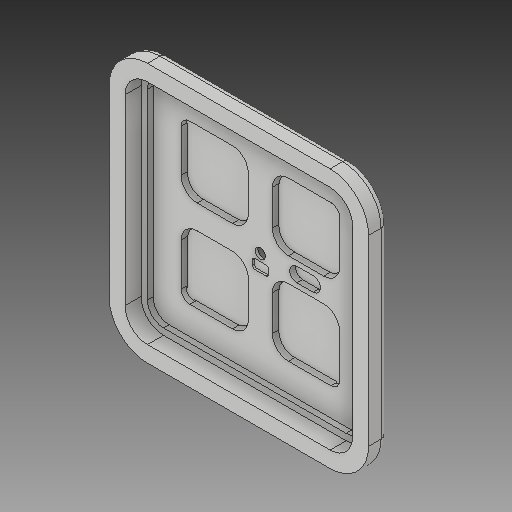
# Autodesk Inventor part: V4
Saved by Autodesk Inventor 2020 (Build 240168000, 168)
## iProperties
Created: 2020-01-08
Part Number: V4
Material: Generic
Document SubType Name: Modeling
Designer: user
Density: 1 g/cm^3
Appearance: Default
Author: user
Autodesk Inventor part; units mm, degrees
ref_plane "YZ Plane" through (0, 0, 0) normal (1, 0, 0) x (0, 1, 0)
ref_plane "XZ Plane" through (0, 0, 0) normal (0, 1, 0) x (-1, 0, 0)
ref_plane "XY Plane" through (0, 0, 0) normal (0, 0, 1) x (1, 0, 0)
sketch "Sketch1" plane through (0, 0, 0) normal (0, 0, 1) x (1, 0, 0)
  line L0 (-28.5, 40.5) -> (28.5, 40.5)
  line L1 (40.5, 28.5) -> (40.5, -28.5)
  line L2 (28.5, -40.5) -> (-28.5, -40.5)
  line L3 (-40.5, -28.5) -> (-40.5, 28.5)
  arc A0 (-28.5, 40.5) -> (-40.5, 28.5) centre (-28.5, 28.5) ccw
  arc A1 (40.5, 28.5) -> (28.5, 40.5) centre (28.5, 28.5) ccw
  arc A2 (28.5, -40.5) -> (40.5, -28.5) centre (28.5, -28.5) ccw
  arc A3 (-40.5, -28.5) -> (-28.5, -40.5) centre (-28.5, -28.5) ccw
  line L4 (-28.5, 28.5) -> (28.5, -28.5) construction
  point P0 (0, 0)
  point P1 (0, 0)
  dimension "d0" = 12
  dimension "d1" = 81
  dimension "d40" = 81
  constraints: 10 end point, 8 point on circle, 8 tangent, 4 centre point, 3 equal radius, 2 parallel, 1 coincident, 1 horizontal, 1 midpoint, 1 perpendicular
  measures "d0" radius of A0
  measures "d1" distance between parallel lines of L2 L0
  measures "d40" distance between parallel lines of L1 L3
extrude "Extrusion1" add sketch "Sketch1" along normal blind 10.25
sketch "Sketch2" plane through (0, 0, 10.25) normal (0, 0, 1) x (1, 0, 0)
  line L0 (28.5, 40.5) -> (-28.5, 40.5) construction
  arc A0 (-28.5, 40.5) -> (-40.5, 28.5) centre (-28.5, 28.5) ccw construction
  line L1 (-40.5, 28.5) -> (-40.5, -28.5) construction
  arc A1 (-40.5, -28.5) -> (-28.5, -40.5) centre (-28.5, -28.5) ccw construction
  line L2 (-28.5, -40.5) -> (28.5, -40.5) construction
  arc A2 (28.5, -40.5) -> (40.5, -28.5) centre (28.5, -28.5) ccw construction
  line L3 (40.5, -28.5) -> (40.5, 28.5) construction
  arc A3 (40.5, 28.5) -> (28.5, 40.5) centre (28.5, 28.5) ccw construction
  line L4 (-28.5, 35.5) -> (28.5, 35.5)
  arc A4 (35.5, 28.5) -> (28.5, 35.5) centre (28.5, 28.5) ccw
  line L5 (35.5, 28.5) -> (35.5, -28.5)
  arc A5 (28.5, -35.5) -> (35.5, -28.5) centre (28.5, -28.5) ccw
  line L6 (28.5, -35.5) -> (-28.5, -35.5)
  arc A6 (-35.5, -28.5) -> (-28.5, -35.5) centre (-28.5, -28.5) ccw
  line L7 (-35.5, -28.5) -> (-35.5, 28.5)
  arc A7 (-28.5, 35.5) -> (-35.5, 28.5) centre (-28.5, 28.5) ccw
  point P0 (0, 0)
  dimension "d4" = 5
  constraints: 8 end point, 8 point on circle, 4 centre point, 7 other
  measures "d4" distance between parallel lines of L1 L7
extrude "Extrusion2" cut sketch "Sketch2" against normal blind 5
sketch "Sketch3" plane through (0, 0, 5.25) normal (0, 0, 1) x (1, 0, 0)
  line L0 (-28.5, 35.5) -> (28.5, 35.5) construction
  arc A0 (-28.5, 35.5) -> (-35.5, 28.5) centre (-28.5, 28.5) ccw construction
  line L1 (-35.5, -28.5) -> (-35.5, 28.5) construction
  arc A1 (-35.5, -28.5) -> (-28.5, -35.5) centre (-28.5, -28.5) ccw construction
  line L2 (28.5, -35.5) -> (-28.5, -35.5) construction
  arc A2 (28.5, -35.5) -> (35.5, -28.5) centre (28.5, -28.5) ccw construction
  line L3 (35.5, 28.5) -> (35.5, -28.5) construction
  arc A3 (35.5, 28.5) -> (28.5, 35.5) centre (28.5, 28.5) ccw construction
  line L4 (28.5, 33.5) -> (-28.5, 33.5)
  arc A4 (-28.5, 33.5) -> (-33.5, 28.5) centre (-28.5, 28.5) ccw
  line L5 (-33.5, 28.5) -> (-33.5, -28.5)
  arc A5 (-33.5, -28.5) -> (-28.5, -33.5) centre (-28.5, -28.5) ccw
  line L6 (-28.5, -33.5) -> (28.5, -33.5)
  arc A6 (28.5, -33.5) -> (33.5, -28.5) centre (28.5, -28.5) ccw
  line L7 (33.5, -28.5) -> (33.5, 28.5)
  arc A7 (33.5, 28.5) -> (28.5, 33.5) centre (28.5, 28.5) ccw
  point P0 (0, 0)
  dimension "d7" = 2
  constraints: 8 end point, 8 point on circle, 4 centre point, 7 other
  measures "d7" distance between parallel lines of L0 L4
extrude "Extrusion3" cut sketch "Sketch3" against normal blind 1.75
chamfer "Chamfer1" distance 9 angle 30 8 edges at (0, 40.5, 0) (36.9853, 36.9853, 0) (40.5, 0, 0) (36.9853, -36.9853, 0) (0, -40.5, 0) (-36.9853, -36.9853, 0) (-40.5, 0, 0) (-36.9853, 36.9853, 0) measured on face at (40, 0, 0) measured on face at (-36.6317, -36.6317, 0) measured on face at (0, 40, 0) measured on face at (0, -40, 0) measured on face at (-36.6317, 36.6317, 0) measured on face at (36.6317, 36.6317, 0) measured on face at (-40, 0, 0) measured on face at (36.6317, -36.6317, 0)
sketch "Sketch5" plane through (0, 0, 0) normal (0, 0, -1) x (-1, 0, 0)
  line L0 (-8.75, 3.75) -> (-19.75, 3.75)
  line L1 (-24.75, 8.75) -> (-24.75, 22.0251)
  line L2 (-22.0251, 24.75) -> (-8.75, 24.75)
  line L3 (-3.75, 19.75) -> (-3.75, 8.75)
  arc A0 (-24.75, 8.75) -> (-19.75, 3.75) centre (-19.75, 8.75) ccw
  arc A1 (-3.75, 19.75) -> (-8.75, 24.75) centre (-8.75, 19.75) ccw
  arc A2 (-8.75, 3.75) -> (-3.75, 8.75) centre (-8.75, 8.75) ccw
  line L4 (17.252, -17.252) -> (-8.75, 8.75) construction
  line L5 (-8.75, 24.25) -> (-22.0251, 24.25)
  line L6 (-24.25, 22.0251) -> (-24.25, 8.75)
  arc A3 (-24.25, 8.75) -> (-19.75, 4.25) centre (-19.75, 8.75) ccw
  line L7 (-19.75, 4.25) -> (-8.75, 4.25)
  arc A4 (-8.75, 4.25) -> (-4.25, 8.75) centre (-8.75, 8.75) ccw
  line L8 (-4.25, 8.75) -> (-4.25, 19.75)
  arc A5 (-4.25, 19.75) -> (-8.75, 24.25) centre (-8.75, 19.75) ccw
  line L9 (-45.752, 45.752) -> (-19.75, 19.75) construction
  line L10 (-8.75, 24.25) -> (-8.75, 4.25) construction
  line L11 (-24.25, 8.75) -> (-4.25, 8.75) construction
  line L12 (-8.75, 24.25) -> (-8.75, 24.75) construction
  line L13 (-24.25, 8.75) -> (-24.75, 8.75) construction
  line L14 (-8.75, 19.75) -> (-19.75, 19.75) construction
  line L15 (-19.75, 8.75) -> (-19.75, 19.75) construction
  arc A6 (-22.2751, 24.5) -> (-22.0251, 24.25) centre (-22.0251, 24.5) ccw
  arc A7 (-22.0251, 24.75) -> (-22.2751, 24.5) centre (-22.0251, 24.5) ccw
  arc A8 (-24.25, 22.0251) -> (-24.5, 21.7751) centre (-24.5, 22.0251) ccw construction
  arc A9 (-24.5, 21.7751) -> (-24.75, 22.0251) centre (-24.5, 22.0251) ccw construction
  line L16 (-23.2626, 23.2626) -> (-22.2019, 24.3232) construction
  line L17 (-23.2626, 23.2626) -> (-24.3232, 22.2019) construction
  arc A10 (-28.5, 31.5) -> (-31.5, 28.5) centre (-28.5, 28.5) ccw construction
  arc A11 (-24.25, 22.0251) -> (-24.75, 22.0251) centre (-24.5, 22.0251) ccw
  line L18 (-3.75, -8.75) -> (-3.75, -19.75)
  line L19 (-8.75, -4.25) -> (-19.75, -4.25)
  line L20 (-4.25, -19.75) -> (-4.25, -8.75)
  line L21 (-24.25, -8.75) -> (-4.25, -8.75) construction
  line L22 (-8.75, -24.25) -> (-8.75, -4.25) construction
  arc A12 (-19.75, -4.25) -> (-24.25, -8.75) centre (-19.75, -8.75) ccw
  line L23 (-8.75, -19.75) -> (-19.75, -19.75) construction
  line L24 (-19.75, -8.75) -> (-19.75, -19.75) construction
  line L25 (-23.2626, -23.2626) -> (-22.2019, -24.3232) construction
  line L26 (-24.25, -8.75) -> (-24.25, -22.0251)
  line L27 (-24.75, -22.0251) -> (-24.75, -8.75)
  line L28 (-24.25, -8.75) -> (-24.75, -8.75) construction
  arc A13 (-19.75, -3.75) -> (-24.75, -8.75) centre (-19.75, -8.75) ccw
  line L29 (-19.75, -3.75) -> (-8.75, -3.75)
  arc A14 (-3.75, -8.75) -> (-8.75, -3.75) centre (-8.75, -8.75) ccw
  arc A15 (-4.25, -8.75) -> (-8.75, -4.25) centre (-8.75, -8.75) ccw
  line L30 (-8.75, -24.75) -> (-22.0251, -24.75)
  line L31 (-22.0251, -24.25) -> (-8.75, -24.25)
  line L32 (-8.75, -24.25) -> (-8.75, -24.75) construction
  arc A16 (-8.75, -24.25) -> (-4.25, -19.75) centre (-8.75, -19.75) ccw
  arc A17 (-8.75, -24.75) -> (-3.75, -19.75) centre (-8.75, -19.75) ccw
  arc A18 (-24.75, -22.0251) -> (-24.5, -22.2751) centre (-24.5, -22.0251) ccw
  arc A19 (-24.5, -22.2751) -> (-24.25, -22.0251) centre (-24.5, -22.0251) ccw
  line L33 (-23.2626, -23.2626) -> (-24.3232, -22.2019) construction
  arc A20 (-21.7751, -24.5) -> (-22.0251, -24.75) centre (-22.0251, -24.5) ccw construction
  arc A21 (-22.0251, -24.25) -> (-21.7751, -24.5) centre (-22.0251, -24.5) ccw construction
  arc A22 (-22.0251, -24.25) -> (-22.0251, -24.75) centre (-22.0251, -24.5) ccw
  line L34 (8.75, -3.75) -> (19.75, -3.75)
  line L35 (4.25, -8.75) -> (4.25, -19.75)
  line L36 (19.75, -4.25) -> (8.75, -4.25)
  line L37 (8.75, -24.25) -> (8.75, -4.25) construction
  line L38 (24.25, -8.75) -> (4.25, -8.75) construction
  arc A23 (4.25, -19.75) -> (8.75, -24.25) centre (8.75, -19.75) ccw
  line L39 (19.75, -8.75) -> (19.75, -19.75) construction
  line L40 (8.75, -19.75) -> (19.75, -19.75) construction
  line L41 (23.2626, -23.2626) -> (24.3232, -22.2019) construction
  line L42 (8.75, -24.25) -> (22.0251, -24.25)
  line L43 (22.0251, -24.75) -> (8.75, -24.75)
  line L44 (8.75, -24.25) -> (8.75, -24.75) construction
  arc A24 (3.75, -19.75) -> (8.75, -24.75) centre (8.75, -19.75) ccw
  line L45 (3.75, -19.75) -> (3.75, -8.75)
  arc A25 (8.75, -3.75) -> (3.75, -8.75) centre (8.75, -8.75) ccw
  arc A26 (8.75, -4.25) -> (4.25, -8.75) centre (8.75, -8.75) ccw
  line L46 (24.75, -8.75) -> (24.75, -22.0251)
  line L47 (24.25, -22.0251) -> (24.25, -8.75)
  line L48 (24.25, -8.75) -> (24.75, -8.75) construction
  arc A27 (24.25, -8.75) -> (19.75, -4.25) centre (19.75, -8.75) ccw
  arc A28 (24.75, -8.75) -> (19.75, -3.75) centre (19.75, -8.75) ccw
  arc A29 (22.0251, -24.75) -> (22.2751, -24.5) centre (22.0251, -24.5) ccw
  arc A30 (22.2751, -24.5) -> (22.0251, -24.25) centre (22.0251, -24.5) ccw
  line L49 (23.2626, -23.2626) -> (22.2019, -24.3232) construction
  arc A31 (24.5, -21.7751) -> (24.75, -22.0251) centre (24.5, -22.0251) ccw construction
  arc A32 (24.25, -22.0251) -> (24.5, -21.7751) centre (24.5, -22.0251) ccw construction
  arc A33 (24.25, -22.0251) -> (24.75, -22.0251) centre (24.5, -22.0251) ccw
  line L50 (3.75, 8.75) -> (3.75, 19.75)
  line L51 (8.75, 4.25) -> (19.75, 4.25)
  line L52 (4.25, 19.75) -> (4.25, 8.75)
  line L53 (24.25, 8.75) -> (4.25, 8.75) construction
  line L54 (8.75, 24.25) -> (8.75, 4.25) construction
  arc A34 (19.75, 4.25) -> (24.25, 8.75) centre (19.75, 8.75) ccw
  line L55 (8.75, 19.75) -> (19.75, 19.75) construction
  line L56 (19.75, 8.75) -> (19.75, 19.75) construction
  line L57 (23.2626, 23.2626) -> (22.2019, 24.3232) construction
  line L58 (24.25, 8.75) -> (24.25, 22.0251)
  line L59 (24.75, 22.0251) -> (24.75, 8.75)
  line L60 (24.25, 8.75) -> (24.75, 8.75) construction
  arc A35 (19.75, 3.75) -> (24.75, 8.75) centre (19.75, 8.75) ccw
  line L61 (19.75, 3.75) -> (8.75, 3.75)
  arc A36 (3.75, 8.75) -> (8.75, 3.75) centre (8.75, 8.75) ccw
  arc A37 (4.25, 8.75) -> (8.75, 4.25) centre (8.75, 8.75) ccw
  line L62 (8.75, 24.75) -> (22.0251, 24.75)
  line L63 (22.0251, 24.25) -> (8.75, 24.25)
  line L64 (8.75, 24.25) -> (8.75, 24.75) construction
  arc A38 (8.75, 24.25) -> (4.25, 19.75) centre (8.75, 19.75) ccw
  arc A39 (8.75, 24.75) -> (3.75, 19.75) centre (8.75, 19.75) ccw
  arc A40 (24.75, 22.0251) -> (24.5, 22.2751) centre (24.5, 22.0251) ccw
  arc A41 (24.5, 22.2751) -> (24.25, 22.0251) centre (24.5, 22.0251) ccw
  line L65 (23.2626, 23.2626) -> (24.3232, 22.2019) construction
  arc A42 (21.7751, 24.5) -> (22.0251, 24.75) centre (22.0251, 24.5) ccw construction
  arc A43 (22.0251, 24.25) -> (21.7751, 24.5) centre (22.0251, 24.5) ccw construction
  arc A44 (22.0251, 24.25) -> (22.0251, 24.75) centre (22.0251, 24.5) ccw
  line L66 (0, 0) -> (0, 0)
  line L67 (24.75, -15.3876) -> (31.5, -15.3876) construction
  line L68 (31.5, 28.5) -> (31.5, -28.5) construction
  line L69 (15.3876, -24.75) -> (15.3876, -31.5) construction
  line L70 (28.5, -31.5) -> (-28.5, -31.5) construction
  point P0 (-22.2751, 24.75)
  point P1 (-24.75, 21.7751)
  point P2 (-24.25, 21.7751)
  point P3 (-22.2751, 24.25)
  point P4 (-24.25, -22.2751)
  point P5 (-24.75, -22.2751)
  point P6 (-21.7751, -24.75)
  point P7 (-21.7751, -24.25)
  point P8 (22.2751, -24.25)
  point P9 (22.2751, -24.75)
  point P10 (24.75, -21.7751)
  point P11 (24.25, -21.7751)
  point P12 (24.25, 22.2751)
  point P13 (24.75, 22.2751)
  point P14 (21.7751, 24.75)
  point P15 (21.7751, 24.25)
  dimension "d23" = 0.5
  dimension "d24" = 5
  dimension "d25" = 20
  dimension "d26" = 0.25
  dimension "d27" = 3
  dimension "d32" = 360
  dimension "d41" = 7.5
  constraints: 138 end point, 96 point on circle, 44 centre point, 27 point on line, 11 tangent, 7 perpendicular, 6 equal length, 4 horizontal, 4 parallel, 3 collinear, 3 equal radius, 2 midpoint, 2 vertical, 1 coincident, 315 other
  measures "d23" distance between parallel lines of L0 L7
  measures "d24" radius of A0
  measures "d25" distance between parallel lines of L8 L6
  measures "d26" radius of A6
  measures "d27" distance of L17.end L16.end
  measures "d41" distance between parallel lines of L50 L3
extrude "Extrusion4" cut sketch "Sketch5" against normal through all
fillet "Fillet2" radius 2 16 edges at (36.9853, 36.9853, 5.1962) (40.5, 0, 5.1962) (36.9853, -36.9853, 5.1962) (0, -40.5, 5.1962) (-36.9853, -36.9853, 5.1962) (-40.5, 0, 5.1962) (-36.9853, 36.9853, 5.1962) (0, 40.5, 5.1962) (-30.6213, 30.6213, 0) (-31.5, 0, 0) (-30.6213, -30.6213, 0) (0, -31.5, 0) (30.6213, -30.6213, 0) (31.5, 0, 0) (30.6213, 30.6213, 0) (0, 31.5, 0)
sketch "Sketch7" plane through (0, 0, 3.5) normal (0, 0, 1) x (1, 0, 0)
  line L0 (-3.75, -8.75) -> (-3.75, -19.75) projected
  arc A0 (-8.75, -24.75) -> (-3.75, -19.75) centre (-8.75, -19.75) ccw projected
  line L1 (-8.75, -24.75) -> (-22.0251, -24.75) projected
  arc A1 (-22.0251, -24.25) -> (-22.0251, -24.75) centre (-22.0251, -24.5) ccw projected
  line L2 (-22.0251, -24.25) -> (-8.75, -24.25) projected
  arc A2 (-8.75, -24.25) -> (-4.25, -19.75) centre (-8.75, -19.75) ccw projected
  line L3 (-4.25, -19.75) -> (-4.25, -8.75) projected
  arc A3 (-4.25, -8.75) -> (-8.75, -4.25) centre (-8.75, -8.75) ccw projected
  line L4 (-8.75, -4.25) -> (-19.75, -4.25) projected
  arc A4 (-19.75, -4.25) -> (-24.25, -8.75) centre (-19.75, -8.75) ccw projected
  line L5 (-24.25, -8.75) -> (-24.25, -22.0251) projected
  arc A5 (-24.75, -22.0251) -> (-24.25, -22.0251) centre (-24.5, -22.0251) ccw projected
  line L6 (-24.75, -22.0251) -> (-24.75, -8.75) projected
  arc A6 (-19.75, -3.75) -> (-24.75, -8.75) centre (-19.75, -8.75) ccw projected
  line L7 (-19.75, -3.75) -> (-8.75, -3.75) projected
  arc A7 (-3.75, -8.75) -> (-8.75, -3.75) centre (-8.75, -8.75) ccw projected
  line L8 (22.0251, 24.25) -> (8.75, 24.25) projected
  arc A8 (8.75, 24.25) -> (4.25, 19.75) centre (8.75, 19.75) ccw projected
  line L9 (4.25, 19.75) -> (4.25, 8.75) projected
  arc A9 (4.25, 8.75) -> (8.75, 4.25) centre (8.75, 8.75) ccw projected
  line L10 (8.75, 4.25) -> (19.75, 4.25) projected
  arc A10 (19.75, 4.25) -> (24.25, 8.75) centre (19.75, 8.75) ccw projected
  line L11 (24.25, 8.75) -> (24.25, 22.0251) projected
  arc A11 (24.75, 22.0251) -> (24.25, 22.0251) centre (24.5, 22.0251) ccw projected
  line L12 (24.75, 22.0251) -> (24.75, 8.75) projected
  arc A12 (19.75, 3.75) -> (24.75, 8.75) centre (19.75, 8.75) ccw projected
  line L13 (19.75, 3.75) -> (8.75, 3.75) projected
  arc A13 (3.75, 8.75) -> (8.75, 3.75) centre (8.75, 8.75) ccw projected
  line L14 (3.75, 8.75) -> (3.75, 19.75) projected
  arc A14 (8.75, 24.75) -> (3.75, 19.75) centre (8.75, 19.75) ccw projected
  line L15 (8.75, 24.75) -> (22.0251, 24.75) projected
  arc A15 (22.0251, 24.25) -> (22.0251, 24.75) centre (22.0251, 24.5) ccw projected
  line L16 (8.75, -3.75) -> (19.75, -3.75) projected
  arc A16 (24.75, -8.75) -> (19.75, -3.75) centre (19.75, -8.75) ccw projected
  line L17 (24.75, -8.75) -> (24.75, -22.0251) projected
  arc A17 (24.25, -22.0251) -> (24.75, -22.0251) centre (24.5, -22.0251) ccw projected
  line L18 (24.25, -22.0251) -> (24.25, -8.75) projected
  arc A18 (24.25, -8.75) -> (19.75, -4.25) centre (19.75, -8.75) ccw projected
  line L19 (19.75, -4.25) -> (8.75, -4.25) projected
  arc A19 (8.75, -4.25) -> (4.25, -8.75) centre (8.75, -8.75) ccw projected
  line L20 (4.25, -8.75) -> (4.25, -19.75) projected
  arc A20 (4.25, -19.75) -> (8.75, -24.25) centre (8.75, -19.75) ccw projected
  line L21 (8.75, -24.25) -> (22.0251, -24.25) projected
  arc A21 (22.0251, -24.75) -> (22.0251, -24.25) centre (22.0251, -24.5) ccw projected
  line L22 (22.0251, -24.75) -> (8.75, -24.75) projected
  arc A22 (3.75, -19.75) -> (8.75, -24.75) centre (8.75, -19.75) ccw projected
  line L23 (3.75, -19.75) -> (3.75, -8.75) projected
  arc A23 (8.75, -3.75) -> (3.75, -8.75) centre (8.75, -8.75) ccw projected
  line L24 (-8.75, 3.75) -> (-19.75, 3.75) projected
  arc A24 (-24.75, 8.75) -> (-19.75, 3.75) centre (-19.75, 8.75) ccw projected
  line L25 (-24.75, 8.75) -> (-24.75, 22.0251) projected
  arc A25 (-24.25, 22.0251) -> (-24.75, 22.0251) centre (-24.5, 22.0251) ccw projected
  line L26 (-24.25, 22.0251) -> (-24.25, 8.75) projected
  arc A26 (-24.25, 8.75) -> (-19.75, 4.25) centre (-19.75, 8.75) ccw projected
  line L27 (-19.75, 4.25) -> (-8.75, 4.25) projected
  arc A27 (-8.75, 4.25) -> (-4.25, 8.75) centre (-8.75, 8.75) ccw projected
  line L28 (-4.25, 8.75) -> (-4.25, 19.75) projected
  arc A28 (-4.25, 19.75) -> (-8.75, 24.25) centre (-8.75, 19.75) ccw projected
  line L29 (-8.75, 24.25) -> (-22.0251, 24.25) projected
  arc A29 (-22.0251, 24.75) -> (-22.0251, 24.25) centre (-22.0251, 24.5) ccw projected
  line L30 (-22.0251, 24.75) -> (-8.75, 24.75) projected
  arc A30 (-3.75, 19.75) -> (-8.75, 24.75) centre (-8.75, 19.75) ccw projected
  line L31 (-3.75, 19.75) -> (-3.75, 8.75) projected
  arc A31 (-8.75, 3.75) -> (-3.75, 8.75) centre (-8.75, 8.75) ccw projected
  line L32 (-28.5, 33.5) -> (28.5, 33.5) projected
  arc A32 (-28.5, 33.5) -> (-33.5, 28.5) centre (-28.5, 28.5) ccw projected
  line L33 (-33.5, -28.5) -> (-33.5, 28.5) projected
  arc A33 (-33.5, -28.5) -> (-28.5, -33.5) centre (-28.5, -28.5) ccw projected
  line L34 (28.5, -33.5) -> (-28.5, -33.5) projected
  arc A34 (28.5, -33.5) -> (33.5, -28.5) centre (28.5, -28.5) ccw projected
  line L35 (33.5, 28.5) -> (33.5, -28.5) projected
  arc A35 (33.5, 28.5) -> (28.5, 33.5) centre (28.5, 28.5) ccw projected
  arc A36 (-24.75, -22.0251) -> (-22.0251, -24.75) centre (-22.0251, -22.0251) ccw
  arc A37 (-22.0251, 24.75) -> (-24.75, 22.0251) centre (-22.0251, 22.0251) ccw
  arc A38 (22.0251, 24.25) -> (22.0251, 24.75) centre (22.0251, 24.5) ccw projected
  arc A39 (24.75, 22.0251) -> (22.0251, 24.75) centre (22.0251, 22.0251) ccw
  line L36 (22.0251, -24.75) -> (8.75, -24.75) projected
  arc A40 (22.0251, -24.75) -> (24.75, -22.0251) centre (22.0251, -22.0251) ccw
  point P0 (0, 0)
  constraints: 8 point on circle, 4 centre point, 4 tangent
extrude "Extrusion6" cut sketch "Sketch7" against normal blind 1.5 contours L0 A0 L1 A1 L2 A2 L3 A3 L4 A4 L5 A5 L6 A6 L7 A7 | A36 A5 L5 A4 L4 A3 L3 A2 L2 A1 | A15 A39 A11 L11 A10 L10 A9 L9 A8 L8 | L8 A8 L9 A9 L10 A10 L11 A11 L12 A12 L13 A13 L14 A14 L15 A15 | L16 A16 L17 A17 L18 A18 L19 A19 L20 A20 L21 A21 L22 A22 L23 A23 | A40 A21 L21 A20 L20 A19 L19 A18 L18 A17 | L24 A24 L25 A25 L26 A26 L27 A27 L28 A28 L29 A29 L30 A30 L31 A31 | A37 A29 L29 A28 L28 A27 L27 A26 L26 A25
sketch "Sketch8" plane through (0, 0, 0) normal (0, 0, -1) x (-1, 0, 0)
  arc A0 (8.75, -4.25) -> (4.25, -8.75) centre (8.75, -8.75) ccw construction
  arc A1 (-8.75, 4.25) -> (-4.25, 8.75) centre (-8.75, 8.75) ccw construction
  line L0 (8.75, -8.75) -> (-8.75, 8.75) construction
  point P0 (0, 0)
  point P1 (0, 0)
  constraints: 2 end point, 1 midpoint
hole "Hole1" at (0, 0, 0) direction (0, 0, 1) diameter 3.2 end through all counterbore diameter 5.7 counterbore depth 2.7
sketch "Sketch10" plane through (0, 0, 3.5) normal (0, 0, 1) x (1, 0, 0)
  line L0 (2.5, -4.461) -> (2.5, -2.961)
  line L1 (1.75, -2.211) -> (-1.75, -2.211)
  line L2 (-2.5, -2.961) -> (-2.5, -4.461)
  line L3 (-1.75, -5.211) -> (1.75, -5.211)
  line L4 (16.4884, 0) -> (11.4084, 0) construction
  line L5 (16.4884, 2.25) -> (11.4084, 2.25)
  line L6 (11.4084, -2.25) -> (16.4884, -2.25)
  arc A0 (16.4884, -2.25) -> (16.4884, 2.25) centre (16.4884, 0) ccw
  arc A1 (11.4084, 2.25) -> (11.4084, -2.25) centre (11.4084, 0) ccw
  circle A2 centre (0, 0) radius 1.6 construction
  line L7 (13.9484, -2.25) -> (13.9484, -3.75) construction
  line L8 (8.75, -3.75) -> (19.75, -3.75) construction
  line L9 (13.9484, 2.25) -> (13.9484, 3.75) construction
  line L10 (8.75, 3.75) -> (19.75, 3.75) construction
  arc A3 (-2.5, -4.461) -> (-1.75, -5.211) centre (-1.75, -4.461) ccw
  arc A4 (1.75, -5.211) -> (2.5, -4.461) centre (1.75, -4.461) ccw
  arc A5 (2.5, -2.961) -> (1.75, -2.211) centre (1.75, -2.961) ccw
  arc A6 (-1.75, -2.211) -> (-2.5, -2.961) centre (-1.75, -2.961) ccw
  line L11 (1.75, -4.461) -> (0, 0) construction
  line L12 (0, 0) -> (-1.75, -4.461) construction
  point P0 (2.5, -5.211)
  point P1 (-2.5, -2.211)
  point P2 (-2.5, -5.211)
  point P3 (13.9484, 0)
  dimension "d70" = 5
  dimension "d71" = 3
  dimension "d73" = 5.08
  dimension "d76" = 0.75
  dimension "d84" = 13.9484
  dimension "d85" = 2.211
  dimension "d86" = 4.5
  constraints: 24 end point, 12 point on circle, 12 tangent, 9 point on line, 6 centre point, 3 equal radius, 3 midpoint, 3 parallel, 2 equal length, 2 horizontal, 2 vertical, 1 coincident, 1 perpendicular
  measures "d70" distance of point (-2.5, -5.211) point (2.5, -5.211)
  measures "d71" distance of point (-2.5, -2.211) point (-2.5, -5.211)
  measures "d73" distance of L5.start L5.end
  measures "d76" radius of A3
  measures "d84" distance of L11.end point (13.948, 0)
  measures "d85" distance from line of L11.end L1
  measures "d86" distance between parallel lines of L5 L6
extrude "Extrusion7" cut sketch "Sketch10" against normal blind 0.64 contours A4 L3 A3 L2 A6 L1 A5 L0
extrude "Extrusion8" cut sketch "Sketch10" against normal blind 1.75 contours A0 L6 A1 L5
sketch "Sketch9" plane through (0, 0, 0) normal (0, 0, -1) x (-1, 0, 0)
  arc A0 (-4.25, 19.75) -> (-8.75, 24.25) centre (-8.75, 19.75) ccw construction
  circle A1 centre (0, 0) radius 1.6 construction
  arc A2 (-24.25, 8.75) -> (-19.75, 4.25) centre (-19.75, 8.75) ccw construction
  line L0 (-8.75, 19.75) -> (-19.75, 8.75) construction
  circle A3 centre (-14.25, 14.25) radius 2
  circle A4 centre (-17.0784, 11.4216) radius 2
  circle A5 centre (-16.25, 10.7859) radius 2
  circle A6 centre (-15.2853, 10.3863) radius 2
  circle A7 centre (-14.25, 10.25) radius 2
  circle A8 centre (-13.2147, 10.3863) radius 2
  circle A9 centre (-12.25, 10.7859) radius 2
  circle A10 centre (-11.4216, 11.4216) radius 2
  circle A11 centre (-10.7859, 12.25) radius 2
  circle A12 centre (-10.3863, 13.2147) radius 2
  circle A13 centre (-10.25, 14.25) radius 2
  circle A14 centre (-10.3863, 15.2853) radius 2
  circle A15 centre (-10.7859, 16.25) radius 2
  circle A16 centre (-11.4216, 17.0784) radius 2
  circle A17 centre (-12.25, 17.7141) radius 2
  circle A18 centre (-13.2147, 18.1137) radius 2
  circle A19 centre (-14.25, 18.25) radius 2
  circle A20 centre (-15.2853, 18.1137) radius 2
  circle A21 centre (-16.25, 17.7141) radius 2
  circle A22 centre (-17.0784, 17.0784) radius 2
  circle A23 centre (-17.7141, 16.25) radius 2
  circle A24 centre (-18.1137, 15.2853) radius 2
  circle A25 centre (-18.25, 14.25) radius 2
  circle A26 centre (-18.1137, 13.2147) radius 2
  circle A27 centre (-17.7141, 12.25) radius 2
  circle A28 centre (-10.7859, -12.25) radius 2
  circle A29 centre (-10.3863, -13.2147) radius 2
  circle A30 centre (-10.3863, -15.2853) radius 2
  circle A31 centre (-10.7859, -16.25) radius 2
  circle A32 centre (-10.25, -14.25) radius 2
  circle A33 centre (-18.1137, -13.2147) radius 2
  circle A34 centre (-18.25, -14.25) radius 2
  circle A35 centre (-18.1137, -15.2853) radius 2
  circle A36 centre (-14.25, -18.25) radius 2
  circle A37 centre (-15.2853, -18.1137) radius 2
  circle A38 centre (-17.7141, -16.25) radius 2
  circle A39 centre (-17.0784, -17.0784) radius 2
  circle A40 centre (-16.25, -17.7141) radius 2
  circle A41 centre (-11.4216, -11.4216) radius 2
  circle A42 centre (-12.25, -10.7859) radius 2
  line L1 (-19.75, -8.75) -> (-8.75, -19.75) construction
  circle A43 centre (-14.25, -14.25) radius 2
  circle A44 centre (-14.25, -10.25) radius 2
  circle A45 centre (-17.7141, -12.25) radius 2
  circle A46 centre (-15.2853, -10.3863) radius 2
  circle A47 centre (-17.0784, -11.4216) radius 2
  circle A48 centre (-16.25, -10.7859) radius 2
  circle A49 centre (-13.2147, -10.3863) radius 2
  circle A50 centre (-11.4216, -17.0784) radius 2
  circle A51 centre (-13.2147, -18.1137) radius 2
  circle A52 centre (-12.25, -17.7141) radius 2
  circle A53 centre (12.25, -10.7859) radius 2
  circle A54 centre (13.2147, -10.3863) radius 2
  circle A55 centre (15.2853, -10.3863) radius 2
  circle A56 centre (16.25, -10.7859) radius 2
  circle A57 centre (14.25, -10.25) radius 2
  circle A58 centre (13.2147, -18.1137) radius 2
  circle A59 centre (14.25, -18.25) radius 2
  circle A60 centre (15.2853, -18.1137) radius 2
  circle A61 centre (18.25, -14.25) radius 2
  circle A62 centre (18.1137, -15.2853) radius 2
  circle A63 centre (16.25, -17.7141) radius 2
  circle A64 centre (17.0784, -17.0784) radius 2
  circle A65 centre (17.7141, -16.25) radius 2
  circle A66 centre (11.4216, -11.4216) radius 2
  circle A67 centre (10.7859, -12.25) radius 2
  line L2 (8.75, -19.75) -> (19.75, -8.75) construction
  circle A68 centre (14.25, -14.25) radius 2
  circle A69 centre (10.25, -14.25) radius 2
  circle A70 centre (12.25, -17.7141) radius 2
  circle A71 centre (10.3863, -15.2853) radius 2
  circle A72 centre (11.4216, -17.0784) radius 2
  circle A73 centre (10.7859, -16.25) radius 2
  circle A74 centre (10.3863, -13.2147) radius 2
  circle A75 centre (17.0784, -11.4216) radius 2
  circle A76 centre (18.1137, -13.2147) radius 2
  circle A77 centre (17.7141, -12.25) radius 2
  circle A78 centre (10.7859, 12.25) radius 2
  circle A79 centre (10.3863, 13.2147) radius 2
  circle A80 centre (10.3863, 15.2853) radius 2
  circle A81 centre (10.7859, 16.25) radius 2
  circle A82 centre (10.25, 14.25) radius 2
  circle A83 centre (18.1137, 13.2147) radius 2
  circle A84 centre (18.25, 14.25) radius 2
  circle A85 centre (18.1137, 15.2853) radius 2
  circle A86 centre (14.25, 18.25) radius 2
  circle A87 centre (15.2853, 18.1137) radius 2
  circle A88 centre (17.7141, 16.25) radius 2
  circle A89 centre (17.0784, 17.0784) radius 2
  circle A90 centre (16.25, 17.7141) radius 2
  circle A91 centre (11.4216, 11.4216) radius 2
  circle A92 centre (12.25, 10.7859) radius 2
  line L3 (19.75, 8.75) -> (8.75, 19.75) construction
  circle A93 centre (14.25, 14.25) radius 2
  circle A94 centre (14.25, 10.25) radius 2
  circle A95 centre (17.7141, 12.25) radius 2
  circle A96 centre (15.2853, 10.3863) radius 2
  circle A97 centre (17.0784, 11.4216) radius 2
  circle A98 centre (16.25, 10.7859) radius 2
  circle A99 centre (13.2147, 10.3863) radius 2
  circle A100 centre (11.4216, 17.0784) radius 2
  circle A101 centre (13.2147, 18.1137) radius 2
  circle A102 centre (12.25, 17.7141) radius 2
  point P0 (0, 0)
  dimension "d58" = 4
  dimension "d61" = 360
  dimension "d65" = 360
  constraints: 101 centre point, 8 end point, 4 point on line, 2 equal radius, 2 point on circle, 1 midpoint, 262 other
  measures "d58" diameter of A3
emboss "Emboss1" sketch "Sketch9" operation add depth 0.5 direction (0, 0, 1) contours A16 A17 A15 | A15 A17 A14 A16 | A14 A17 A13 A16 | A10 A11 A9 | A10 A12 A9 A11 | A10 A13 A9 A12 | A13 A16 | A10 A13 | A16 A18 A15 A17 | A15 A18 A14 A17 | A14 A17 | A9 A11 A8 A10 | A9 A12 A8 A11 | A9 A12 | A17 A14 A16 A13 | A13 A10 A12 A9 | A16 A19 A15 A18 | A15 A18 | A18 A15 A17 A14 | A8 A11 A7 A10 | A8 A11 | A12 A9 A11 A8 | A17 A15 A16 A14 | A12 A10 A11 A9 | A16 A19 | A19 A16 A18 A15 | A7 A10 | A11 A8 A10 A7 | A18 A16 A17 A15 | A11 A9 A10 A8 | A17 A16 A15 | A11 A10 A9 | A22 A23 A21 | A21 A23 A20 A22 | A20 A23 A19 A22 | A19 A22 | A4 A5 A27 | A4 A6 A27 A5 | A4 A7 A27 A6 | A4 A7 | A22 A24 A21 A23 | A21 A24 A20 A23 | A20 A23 | A23 A20 A22 A19 | A27 A5 A26 A4 | A27 A6 A26 A5 | A27 A6 | A7 A4 A6 A27 | A22 A25 A21 A24 | A21 A24 | A24 A21 A23 A20 | A23 A21 A22 A20 | A26 A5 A25 A4 | A26 A5 | A6 A27 A5 A26 | A6 A4 A5 A27 | A22 A25 | A25 A22 A24 A21 | A24 A22 A23 A21 | A23 A22 A21 | A25 A4 | A5 A26 A4 A25 | A5 A27 A4 A26 | A5 A4 A27 | A44 A41 | A41 A46 A42 A44 | A42 A46 A49 A44 | A49 A46 A44 | A44 A42 A46 A41 | A46 A42 | A42 A48 A49 A46 | A46 A49 A48 A44 | A44 A49 A46 A42 | A46 A49 A48 A42 | A48 A49 | A48 A49 A47 A44 | A44 A46 A49 | A46 A44 A48 A49 | A48 A44 A47 A49 | A47 A44 | A36 A50 | A36 A52 A37 A50 | A51 A37 A52 A36 | A36 A37 A51 | A36 A51 A37 | A36 A52 A37 A51 | A36 A50 A37 A52 | A37 A52 | A36 A40 A51 A37 | A51 A40 A52 A37 | A37 A51 A40 A36 | A37 A52 A40 A51 | A36 A39 A51 A40 | A51 A40 | A40 A51 A39 A36 | A36 A39 | A68 | A78 A99 | A78 A99 A91 A94 | A99 A79 A92 A78 | A78 A92 A91 A99 | A94 A91 A99 A78 | A94 A91 | A99 A92 A94 A91 | A91 A92 A99 | A99 A78 A92 A79 | A79 A92 | A99 A91 A92 A78 | A94 A92 A96 A91 | A94 A92 A99 A91 | A91 A96 A92 A94 | A99 A92 A91 | A96 A92 | A102 A80 | A102 A80 A101 A81 | A81 A101 A100 A102 | A102 A100 A101 | A102 A81 A101 A80 | A102 A100 A101 A81 | A102 A101 A100 | A101 A81 | A81 A86 A100 A101 | A101 A100 A86 A102 | A84 A85 A83 | A83 A85 A95 A84 | A95 A85 A97 A84 | A97 A84 | A101 A100 A86 A81 | A101 A102 A86 A100 | A97 A85 A95 A84 | A84 A95 A85 A83 | A83 A85 A84 | A86 A100 A87 A102 | A86 A100 | A85 A84 A88 A83 | A83 A88 A95 A85 | A95 A85 | A86 A102 A87 A100 | A85 A95 A88 A83 | A83 A88 A84 A85 | A87 A102 | A88 A84 A89 A83 | A83 A88 | A83 A89 A84 A88 | A89 A84
equation "\"d40\" = d1"
equation "\"d26\" = 0.5 * d23"
body "Solid1"
